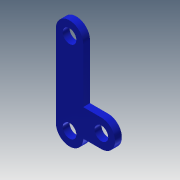
# Autodesk Inventor part: tahlo3
Saved by Autodesk Inventor 2013 (Build 170138000, 138)
## iProperties
Created: 2013-02-09
Part Number: tahlo3
Material: Generic
Document SubType Name: Modeling
Designer: idle-rug
Density: 1 g/cm^3
Author: idle-rug
Autodesk Inventor part; units mm, degrees
ref_plane "YZ Plane" through (0, 0, 0) normal (1, 0, 0) x (0, 1, 0)
ref_plane "XZ Plane" through (0, 0, 0) normal (0, 1, 0) x (-1, 0, 0)
ref_plane "XY Plane" through (0, 0, 0) normal (0, 0, 1) x (1, 0, 0)
sketch "Sketch1" plane through (0, 0, 0) normal (0, 1, 0) x (-1, 0, 0)
  line L0 (3, 9) -> (-3, 9)
  line L1 (-3, 9) -> (-3, -9)
  line L2 (-3, -9) -> (3, -9)
  line L3 (3, -9) -> (3, 9)
  line L4 (3, 9) -> (-3, -9) construction
  line L5 (-3, 9) -> (3, -9) construction
  circle A0 centre (0, 9) radius 3
  circle A1 centre (0, -9) radius 3
  line L6 (-3, -9) -> (-7, -9)
  line L7 (-7, -9) -> (-7, -5)
  line L8 (-7, -5) -> (-7, -3)
  line L9 (-7, -3) -> (-3, -3)
  line L10 (-7, -3) -> (-7, -6)
  circle A2 centre (-7, -6) radius 3
  line L11 (-3, -3) -> (-3, -9)
  point P0 (0, 0)
  dimension "d0" = 6
  dimension "d1" = 18
  dimension "d2" = 6
  dimension "d4" = 6
  dimension "d5" = 4
  dimension "d6" = 4
  dimension "d7" = 2
  dimension "d10" = 3
  dimension "d11" = 6
  constraints: 24 end point, 4 midpoint, 4 perpendicular, 3 centre point, 3 parallel, 3 point on line, 1 coincident, 1 horizontal
  measures "d0" distance of L2.end L1.end
  measures "d1" distance of L1.end L0.end
  measures "d2" diameter of A0
  measures "d4" diameter of A1
  measures "d5" distance of L1.end L6.end
  measures "d6" distance of L6.end L7.end
  measures "d7" distance of L7.end L8.end
  measures "d10" distance of L8.end L10.end
  measures "d11" diameter of A2
extrude "Extrusion1" add sketch "Sketch1" along normal blind 1.5 contours A0 L0 | L0 A0 | L3 A1 L1 A0 | A1 L2 | L2 A1 | A2 L7 L8 | L8 L7 A2
sketch "Sketch2" plane through (0, 1.5, 0) normal (0, 1, 0) x (1, 0, 0)
  line L0 (3, -9) -> (3, 9) projected
  arc A0 (3, 9) -> (-3, 9) centre (0, 9) ccw projected
  line L1 (-3, 9) -> (-3, -9) projected
  arc A1 (-3, -9) -> (3, -9) centre (0, -9) ccw projected
  circle A2 centre (0, 9) radius 1.5
  circle A3 centre (0, -9) radius 1.5
  line L2 (3, 9) -> (7, 9)
  line L3 (7, 9) -> (7, 3)
  line L4 (7, 3) -> (3, 3)
  line L5 (3, 3) -> (3, 9)
  point P0 (0, 0)
  dimension "d14" = 3
  dimension "d15" = 3
  dimension "d16" = 4
  dimension "d17" = 6
  constraints: 8 end point, 3 perpendicular, 2 centre point, 2 coincident, 1 collinear, 1 point on line, 1 tangent
  measures "d14" diameter of A2
  measures "d15" diameter of A3
  measures "d16" distance of L0.end L2.end
  measures "d17" distance of L2.end L3.end
extrude "Extrusion2" cut sketch "Sketch2" against normal blind 1.5 contours L0 L2 L3 L4 | A2 | A3
sketch "Sketch3" plane through (0, 1.5, 0) normal (0, 1, 0) x (1, 0, 0)
  line L0 (3, -9) -> (3, 9) projected
  arc A0 (3, 9) -> (-3, 9) centre (0, 9) ccw projected
  line L1 (-3, 9) -> (-3, -9) projected
  line L2 (3, 9) -> (7, 9)
  line L3 (7, 9) -> (7, 3)
  line L4 (7, 3) -> (3, 3)
  line L5 (3, 3) -> (3, 9)
  point P0 (0, 0)
  dimension "d20" = 4
  dimension "d21" = 6
  dimension "d22" = 4
  constraints: 8 end point, 2 perpendicular, 1 collinear, 1 point on line, 1 tangent
  measures "d20" distance of L0.end L2.end
  measures "d21" distance of L2.end L3.end
  measures "d22" distance of L3.end L4.end
extrude "Extrusion3" add sketch "Sketch3" against normal blind 1.5
sketch "Sketch4" plane through (0, 1.5, 0) normal (0, 1, 0) x (1, 0, 0)
  arc A0 (7, 3) -> (7, 9) centre (7, 6) ccw projected
  circle A1 centre (7, 6) radius 1.5
  point P0 (0, 0)
  dimension "d25" = 3
  constraints: 1 centre point, 1 coincident
  measures "d25" diameter of A1
extrude "Extrusion4" cut sketch "Sketch4" against normal blind 1.5
sketch "Sketch5" plane through (0, 0, 0) normal (0, -1, 0) x (1, 0, 0)
  circle A0 centre (7, -6) radius 1.5 projected
  circle A1 centre (0, 9) radius 1.5 projected
  circle A2 centre (0, -9) radius 1.5 projected
  arc A3 (7, -9) -> (7, -3) centre (7, -6) ccw projected
  arc A4 (3, 9) -> (-3, 9) centre (0, 9) ccw projected
  arc A5 (-3, -9) -> (3, -9) centre (0, -9) ccw projected
  circle A6 centre (0, 9) radius 0.1
  circle A7 centre (0, -9) radius 0.1
  circle A8 centre (7, -6) radius 0.1
  point P0 (0, 0)
  dimension "d28" = 0.2
  dimension "d29" = 0.2
  dimension "d30" = 0.2
  constraints: 3 centre point, 3 coincident
  measures "d28" diameter of A6
  measures "d29" diameter of A7
  measures "d30" diameter of A8
extrude "Extrusion5" add sketch "Sketch5" against normal blind 1.5
sketch "Sketch6" plane through (0, 0, 0) normal (0, -1, 0) x (1, 0, 0)
  circle A0 centre (0, -9) radius 0.1 projected
  circle A1 centre (7, -6) radius 0.1 projected
  circle A2 centre (0, 9) radius 0.1 projected
  arc A3 (7, -9) -> (7, -3) centre (7, -6) ccw projected
  arc A4 (3, 9) -> (-3, 9) centre (0, 9) ccw projected
  arc A5 (-3, -9) -> (3, -9) centre (0, -9) ccw projected
  circle A6 centre (0, 9) radius 1.5
  circle A7 centre (0, -9) radius 1.5
  circle A8 centre (7, -6) radius 1.5
  point P0 (0, 0)
  dimension "d33" = 3
  dimension "d34" = 3
  dimension "d35" = 3
  constraints: 3 centre point, 3 coincident
  measures "d33" diameter of A6
  measures "d34" diameter of A7
  measures "d35" diameter of A8
extrude "Extrusion6" cut sketch "Sketch6" against normal blind 2
sketch "Sketch7" plane through (0, 0, 0) normal (0, -1, 0) x (1, 0, 0)
  arc A0 (-3, -9) -> (3, -9) centre (0, -9) ccw projected
  line L0 (3, -9) -> (7, -9) projected
  line L1 (0, -9) -> (0, -5)
  circle A1 centre (0, -5) radius 1.5
  point P0 (0, 0)
  dimension "d38" = 4
  dimension "d39" = 3
  constraints: 2 end point, 1 centre point, 1 coincident, 1 perpendicular
  measures "d38" distance of L1.start L1.end
  measures "d39" diameter of A1
extrude "Extrusion7" cut sketch "Sketch7" against normal blind 2
sketch "Sketch8" plane through (0, 0, 0) normal (0, -1, 0) x (1, 0, 0)
  circle A0 centre (0, -5) radius 1.5 projected
  point P0 (0, 0)
extrude "Extrusion8" add sketch "Sketch8" against normal blind 2
body "Solid1"
